# Autodesk Inventor part: 3V
Saved by Autodesk Inventor 2016 (Build 200138000, 138)
## iProperties
Created: 2016-04-08
Part Number: 3V
Material: Generic
Document SubType Name: Modeling
Designer: Paschalis
Density: 1 g/cm^3
Appearance: BATTCON_12MM, 3V
Author: Paschalis
Autodesk Inventor part; units mm, degrees
ref_plane "YZ Plane" through (0, 0, 0) normal (1, 0, 0) x (0, 1, 0)
ref_plane "XZ Plane" through (0, 0, 0) normal (0, 1, 0) x (-1, 0, 0)
ref_plane "XY Plane" through (0, 0, 0) normal (0, 0, 1) x (1, 0, 0)
sketch "BATTCON_12MM, 3V_13" plane through (0, 0, 0) normal (0, 0, 1) x (1, 0, 0)
  line L0 (-6.1976, 6.0635) -> (6.096, 6.0635)
  line L1 (6.096, 6.0635) -> (6.096, -6.35)
  line L2 (6.096, -6.35) -> (-6.1976, -6.35)
  line L3 (-6.1976, -6.35) -> (-6.1976, 6.0635)
  constraints: 8 end point
extrude "Extrusion1" add sketch "BATTCON_12MM, 3V_13" along normal blind 1
body "Solid1"
